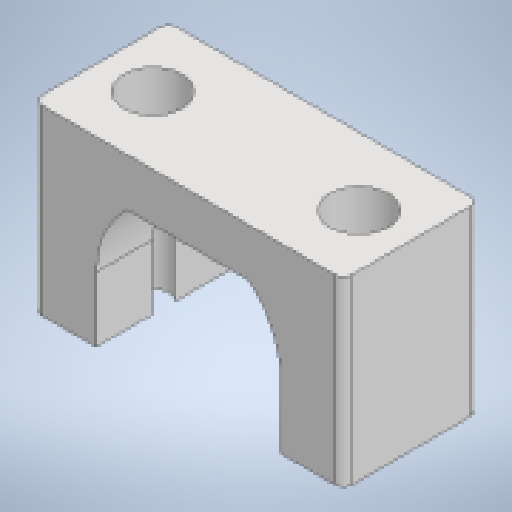
# Autodesk Inventor part: Large Drive Motors Mount Cap
Saved by Autodesk Inventor 2023 (Build 270158000, 158)
## iProperties
Created: 2024-10-28
Part Number: Large Drive Motors Mount Cap
Material: Generic
Document SubType Name: Modeling
Designer: Ethan
Density: 1 g/cm^3
Appearance: Default
Author: Ethan
Autodesk Inventor part; units mm, degrees
ref_plane "YZ Plane" through (0, 0, 0) normal (1, 0, 0) x (0, 1, 0)
ref_plane "XZ Plane" through (0, 0, 0) normal (0, 1, 0) x (-1, 0, 0)
ref_plane "XY Plane" through (0, 0, 0) normal (0, 0, 1) x (1, 0, 0)
sketch "Mount Shape Sketch" plane through (0, 0, 0) normal (0, 0, 1) x (1, 0, 0)
  circle A0 centre (0, 0) radius 8.115
  line L0 (-5.4362, 6.025) -> (5.4362, 6.025)
  line L1 (-5.4362, -6.025) -> (5.4362, -6.025)
  line L2 (-8.115, 0) -> (-8.115, -5.525)
  line L3 (8.115, 0) -> (8.115, -5.525)
  line L4 (8.115, -5.525) -> (15, -5.525)
  line L5 (15, -5.525) -> (15, 12.9873)
  line L6 (15, 12.9873) -> (-15, 12.9873)
  line L7 (-15, 12.9873) -> (-15, -5.525)
  line L8 (-15, -5.525) -> (-8.115, -5.525)
  line L9 (0, 17.2077) -> (0, -12.3355) construction
  dimension "d0" = 16.23
  dimension "d1" = 12.05
  dimension "d3" = 30
  dimension "d15" = 12.9873
  dimension "d18" = 0.5
  constraints: 18 end point, 6 point on circle, 4 perpendicular, 2 horizontal, 2 parallel, 1 centre point, 1 coincident, 1 collinear, 1 tangent, 1 vertical, 2 other
  measures "d0" diameter of A0
  measures "d1" distance between parallel lines of L0 L1
  measures "d3" distance of L5.end L6.end
  measures "d15" distance from line of point (0, 0) L6
  measures "d18" distance between parallel lines of L4 L1
extrude "Mount Shape" add sketch "Mount Shape Sketch" along normal mid plane 15 contours A0 L2 L8 L7 L6 L5 L4 L3 | L0 A0
sketch "Sketch2" plane through (-15, 12.9873, 7.5) normal (0, 1, 0) x (1, 0, 0)
  circle A0 centre (3.585, 7.5) radius 1.75
  line L0 (20.4362, 15) -> (9.5638, 15) construction
  line L1 (15, 15) -> (15, 0) construction
  line L2 (30, 0) -> (0, 0) construction
  line L3 (15, 7.5) -> (3.585, 7.5) construction
  circle A1 centre (26.415, 7.5) radius 1.75
  dimension "d6" = 3.5
  dimension "d7" = 11.415
  dimension "d14" = 22.83
  constraints: 4 end point, 2 centre point, 2 midpoint, 1 coincident, 1 horizontal, 1 symmetric about line, 1 other
  measures "d6" diameter of A0
  measures "d7" distance from line of L1 A0.centre
  measures "d14" distance of A1.centre A0.centre
extrude "Screw Shaft Holes" cut sketch "Sketch2" against normal through all
sketch "Sketch3" plane through (-15, 12.9873, 7.5) normal (0, 1, 0) x (1, 0, 0)
  circle A0 centre (3.585, 7.5) radius 1.75 projected
  circle A1 centre (3.585, 7.5) radius 3.25
  circle A2 centre (26.415, 7.5) radius 3.25
  circle A3 centre (26.415, 7.5) radius 1.75 projected
  point P0 (15, 7.5)
  dimension "d10" = 6.5
  constraints: 2 centre point, 1 coincident, 1 concentric, 1 equal radius
  measures "d10" diameter of A1
extrude "Screw Head Holes" cut sketch "Sketch3" against normal blind 6.8 contours A0 | A1 | A2 | A3
fillet "Outer Fillet" radius 1 4 edges at (15, 3.7311, -7.5) (15, 3.7311, 7.5) (-15, 3.7311, 7.5) (-15, 3.7311, -7.5)
body "Solid1"
